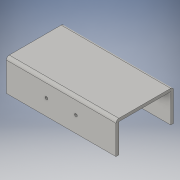
# Autodesk Inventor part: track bracket
Saved by Autodesk Inventor 2016 (Build 200138000, 138)
## iProperties
Created: 2015-10-30
Part Number: track bracket
Material: Generic
Document SubType Name: Modeling
Designer: RoboticsUser
Density: 1 g/cm^3
Appearance: Default
Author: RoboticsUser
Autodesk Inventor part; units mm, degrees
ref_plane "YZ Plane" through (0, 0, 0) normal (1, 0, 0) x (0, 1, 0)
ref_plane "XZ Plane" through (0, 0, 0) normal (0, 1, 0) x (-1, 0, 0)
ref_plane "XY Plane" through (0, 0, 0) normal (0, 0, 1) x (1, 0, 0)
sketch "Sketch1" plane through (0, 0, 0) normal (0, 1, 0) x (-1, 0, 0)
  line L0 (0, 0) -> (-120.65, 0)
  line L1 (-120.65, 0) -> (-120.65, -63.5)
  line L2 (-120.65, -63.5) -> (0, -63.5)
  line L3 (0, -63.5) -> (0, 0)
  dimension "d0" = 120.65
  dimension "d1" = 63.5
  constraints: 8 end point, 2 parallel, 1 horizontal, 1 perpendicular
  measures "d0" distance of L2.end L1.end
  measures "d1" distance of L1.end L0.end
extrude "Extrusion1" add sketch "Sketch1" along normal blind 3.175
sketch "Sketch2" plane through (0, 0, 0) normal (0, 0, 1) x (1, 0, 0)
  line L0 (0, 0) -> (120.65, 0) projected
  line L1 (0, 0) -> (120.65, 0)
  line L2 (120.65, 0) -> (120.65, -31.75)
  line L3 (120.65, -31.75) -> (0, -31.75)
  line L4 (0, -31.75) -> (0, 0)
  dimension "d4" = 31.75
  constraints: 8 end point, 2 parallel, 1 horizontal, 1 perpendicular
  measures "d4" distance of L1.end L2.end
extrude "Extrusion2" add sketch "Sketch2" against normal blind 3.175
sketch "Sketch4" plane through (120.65, 0, -63.5) normal (0, 0, -1) x (-1, 0, 0)
  line L0 (0, -31.75) -> (0, 3.175) projected
  line L1 (120.65, -31.75) -> (120.65, 3.175) projected
  line L2 (0, 3.175) -> (120.65, 3.175)
  line L3 (120.65, 3.175) -> (120.65, -31.75)
  line L4 (120.65, -31.75) -> (0, -31.75)
  line L5 (0, -31.75) -> (0, 3.175)
  point P0 (120.65, 0)
  constraints: 8 end point, 2 parallel, 1 horizontal, 1 perpendicular
extrude "Extrusion4" add sketch "Sketch4" against normal blind 3.175
fillet "Fillet1" radius 3.175 1 edges at (60.325, 3.175, 0)
fillet "Fillet2" radius 3.175 1 edges at (60.325, 3.175, -63.5)
sketch "Sketch5" plane through (0, -31.75, 0) normal (0, 0, 1) x (1, 0, 0)
  line L0 (120.65, 0) -> (0, 0) projected
  line L1 (120.65, 34.925) -> (0, 34.925) projected
  line L2 (120.65, 0) -> (120.65, 31.75) projected
  line L3 (0, 0) -> (0, 31.75) projected
  point P0 (44.069, 17.4625)
  point P1 (76.581, 17.4625)
  point P2 (60.325, 17.4625)
  dimension "d14" = 32.512
  dimension "d15" = 34.925
  dimension "d16" = 17.4625
  dimension "d17" = 17.4625
  dimension "d18" = 120.65
  dimension "d20" = 16.256
  dimension "d21" = 17.4625
  dimension "d22" = 60.325
  dimension "d23" = 16.256
  measures "d14" distance of point (44.069, 17.462) point (76.581, 17.462)
  measures "d15" distance between parallel lines of L1 L0
  measures "d16" distance from line of L0 point (44.069, 17.462)
  measures "d17" distance from line of point (76.581, 17.462) L0
  measures "d18" distance between parallel lines of L2 L3
  measures "d20" distance of point (60.325, 17.462) point (44.069, 17.462)
  measures "d21" distance from line of L0 point (60.325, 17.462)
  measures "d22" distance from line of point (60.325, 17.462) L2
  measures "d23" distance of point (60.325, 17.462) point (76.581, 17.462)
hole "Hole1" at (44.069, -14.2875, 0) at (76.581, -14.2875, 0) direction (0, 0, -1) diameter 3.0625 end through all
equation "\"d16\" = 0.5 * d15"
equation "\"d17\" = d16"
equation "\"d20\" = 0.5 * d14"
equation "\"d21\" = d16"
equation "\"d22\" = 0.5 * d18"
body "Solid1"
